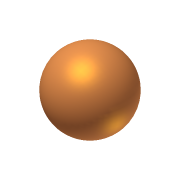
# Autodesk Inventor part: Ball
Saved by Autodesk Inventor 2012 (Build 160160000, 160)
## iProperties
Created: 2012-01-13
Part Number: Ball
Material: Wood (Birch)
Document SubType Name: Modeling
Designer: JesseK
Density: 0.55 g/cm^3
Mass: 17.8507 g
Surface Area: 2555.58 cm^2
Volume: 32.4558 cm^3
Author: JesseK
Autodesk Inventor part; units mm, degrees
ref_plane "YZ Plane" through (0, 0, 0) normal (1, 0, 0) x (0, 1, 0)
ref_plane "XZ Plane" through (0, 0, 0) normal (0, 1, 0) x (-1, 0, 0)
ref_plane "XY Plane" through (0, 0, 0) normal (0, 0, 1) x (1, 0, 0)
sketch "Sketch1" plane through (0, 0, 0) normal (0, 0, 1) x (1, 0, 0)
  arc A0 (0, 100.965) -> (0, -100.965) centre (0, 0) ccw
  arc A1 (0, 100.711) -> (0, -100.711) centre (0, 0) ccw
  line L0 (0, 100.965) -> (0, 100.711)
  line L1 (0, -100.711) -> (0, -100.965)
  dimension "d0" = 100.965
  dimension "d2" = 0.254
  constraints: 4 end point, 4 point on circle, 2 centre point, 2 coincident, 2 vertical
  measures "d0" radius of A0
  measures "d2" radial gap between concentric circles of A0 A1
revolve "Revolution2" add sketch "Sketch1" angle 360 about axis through (0, 100.965, 0) along (0, -1, 0)
body "Solid2"
